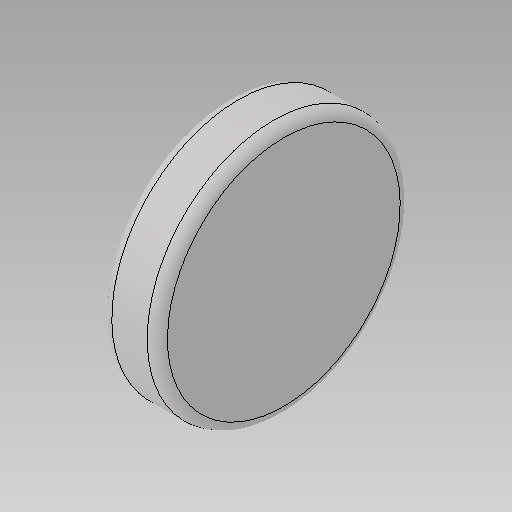
# Autodesk Inventor part: Axle_collar
Saved by Autodesk Inventor 2020 (Build 240168000, 168)
## iProperties
Created: 2019-02-05
Part Number: Axle_collar
Material: Generic
Document SubType Name: Modeling
Designer: Varga Daniel
Density: 1 g/cm^3
Appearance: Default
Author: Varga Daniel
Autodesk Inventor part; units mm, degrees
ref_plane "YZ Plane" through (0, 0, 0) normal (1, 0, 0) x (0, 1, 0)
ref_plane "XZ Plane" through (0, 0, 0) normal (0, 1, 0) x (-1, 0, 0)
ref_plane "XY Plane" through (0, 0, 0) normal (0, 0, 1) x (1, 0, 0)
derived "Connector_pin_base.ipt"
sketch "Pin_base_sketch" plane through (0, 0, 0) normal (0, 0, 1) x (1, 0, 0)
  line L0 (0, 0) -> (23.0918, 0) construction
  line L1 (0, 0) -> (0, 6.22) construction
  line L2 (0, 3.75) -> (0.525, 3.75)
  line L3 (0.825, 3.45) -> (0.825, 2.4)
  line L4 (0.825, 2.4) -> (9.225, 2.4)
  line L5 (0, 0) -> (0, 3.75)
  line L6 (0, 0) -> (3.25, 0)
  arc A0 (0.825, 3.45) -> (0.525, 3.75) centre (0.525, 3.45) ccw
  line L7 (0.825, 2.4) -> (0.825, 0.575)
  line L8 (0, 0) -> (-23.0918, 0) construction
  line L9 (9.225, 2.4) -> (9.225, 0.575)
  line L10 (10.025, 2.4) -> (10.025, 2.1865) construction
  line L11 (9.225, 2.4) -> (10.025, 2.4) construction
  line L12 (9.625, 2.4) -> (9.625, 0) construction
  line L13 (10.1291, 2.615) -> (7.4184, 2.615) construction
  line L14 (10.025, 0.575) -> (9.225, 0.575) construction
  line L15 (10.025, 0.575) -> (10.025, 0)
  arc A1 (7.1, 0.575) -> (6.525, 0) centre (7.1, 0) ccw construction
  line L16 (9.225, 0.575) -> (7.1, 0.575) construction
  line L17 (9.225, 0.575) -> (9.225, 0)
  line L18 (0, 0.575) -> (0.825, 0.575) construction
  arc A2 (3.25, 0) -> (2.675, 0.575) centre (2.675, 0) ccw construction
  line L19 (0.825, 0.575) -> (0.825, 0)
  line L20 (0.825, 0.575) -> (2.675, 0.575) construction
  line L21 (0, 0) -> (-3.25, 0)
  line L22 (0, 3.75) -> (-0.525, 3.75)
  line L23 (-0.825, 3.45) -> (-0.825, 2.4)
  arc A3 (-0.525, 3.75) -> (-0.825, 3.45) centre (-0.525, 3.45) ccw
  line L24 (-0.825, 2.4) -> (-0.825, 0.575)
  line L25 (-0.825, 0.575) -> (-0.825, 0)
  line L26 (0, 0.575) -> (-0.825, 0.575) construction
  line L27 (-0.825, 2.4) -> (-9.225, 2.4)
  line L28 (-9.225, 2.4) -> (-9.225, 0)
  line L29 (-10.875, 2.4) -> (-10.875, 0)
  line L30 (-10.5179, 2.55) -> (-9.5821, 2.55)
  line L31 (-10.05, 2.55) -> (-10.05, 0) construction
  line L32 (-9.225, 2.4) -> (-10.875, 2.4) construction
  arc A4 (-10.5179, 2.55) -> (-10.875, 2.4) centre (-10.5179, 2.05) ccw
  arc A5 (-9.225, 2.4) -> (-9.5821, 2.55) centre (-9.5821, 2.05) ccw
  line L33 (-10.875, 2.4) -> (-19.275, 2.4)
  line L34 (-19.275, 2.4) -> (-19.275, 0)
  line L35 (-19.275, 0) -> (-16.575, 0)
  line L36 (-19.275, 2.4) -> (-20.075, 2.4) construction
  line L37 (-20.075, 2.4) -> (-20.075, 2.1865) construction
  line L38 (-20.075, 0) -> (-19.275, 0)
  line L39 (-19.675, 2.4) -> (-19.675, 0) construction
  line L40 (-19.6465, 2.615) -> (-17.4324, 2.615) construction
  line L41 (-0.825, 0.575) -> (-2.675, 0.575) construction
  arc A6 (-2.675, 0.575) -> (-3.25, 0) centre (-2.675, 0) ccw construction
  line L42 (-12.725, 0.575) -> (-7.375, 0.575) construction
  arc A7 (-6.8, 0) -> (-7.375, 0.575) centre (-7.375, 0) ccw construction
  arc A8 (-12.725, 0.575) -> (-13.3, 0) centre (-12.725, 0) ccw construction
  line L43 (-20.075, 0.575) -> (-17.15, 0.575) construction
  arc A9 (-16.575, 0) -> (-17.15, 0.575) centre (-17.15, 0) ccw construction
  line L44 (-16.575, 0) -> (-13.3, 0)
  line L45 (-20.075, 0.575) -> (-20.075, 0)
  line L46 (-13.3, 0) -> (-10.875, 0)
  line L47 (-6.8, 0) -> (-10.875, 0)
  line L48 (-3.25, 0) -> (-6.8, 0)
  line L49 (3.25, 0) -> (6.525, 0)
  line L50 (6.525, 0) -> (10.025, 0)
  arc A10 (-17.15, -0.575) -> (-16.575, 0) centre (-17.15, 0) ccw construction
  line L51 (-20.075, -0.575) -> (-20.075, 0) construction
  line L52 (-20.075, -0.575) -> (-17.15, -0.575) construction
  line L53 (-12.725, -0.575) -> (-7.375, -0.575) construction
  arc A11 (-13.3, 0) -> (-12.725, -0.575) centre (-12.725, 0) ccw construction
  arc A12 (-7.375, -0.575) -> (-6.8, 0) centre (-7.375, 0) ccw construction
  arc A13 (-3.25, 0) -> (-2.675, -0.575) centre (-2.675, 0) ccw construction
  line L54 (-0.825, -0.575) -> (-2.675, -0.575) construction
  line L55 (0, -0.575) -> (-0.825, -0.575) construction
  line L56 (0, -0.575) -> (0.825, -0.575) construction
  line L57 (0.825, -0.575) -> (2.675, -0.575) construction
  arc A14 (2.675, -0.575) -> (3.25, 0) centre (2.675, 0) ccw construction
  arc A15 (6.525, 0) -> (7.1, -0.575) centre (7.1, 0) ccw construction
  line L58 (9.225, -0.575) -> (7.1, -0.575) construction
  line L59 (10.025, -0.575) -> (9.225, -0.575) construction
  line L60 (10.025, -0.575) -> (10.025, 0) construction
  line L61 (-0.025, 0) -> (-0.025, 4.3146) construction
  line L62 (0.025, 0) -> (0.025, 4.3146) construction
  line L63 (-10.075, 0) -> (-10.075, 4.2477) construction
  line L64 (-10.025, 0) -> (-10.025, 4.2339) construction
  arc A16 (-19.275, 2.4) -> (-20.075, 2.1865) centre (-19.6465, 2.1865) ccw
  line L65 (-20.075, 2.1865) -> (-20.075, 0.575)
  arc A17 (10.025, 2.1865) -> (9.225, 2.4) centre (9.5965, 2.1865) ccw
  line L66 (10.025, 2.1865) -> (10.025, 0.575)
revolve "Revolution2" add sketch "Pin_base_sketch" angle 360 about axis through (0, 0, 0) along (1, 0, 0) contours L2 A0 L3 L7 L19 L6 L5 | L5 L21 L25 L24 L23 A3 L22
equation "\"Axle_collar_thickness\" = 1.8"
body "Solid2"
